Autodesk Inventor part; units mm, degrees
(part 4 of 6)
  line L2686 (41.0698, 0.537) -> (41.0192, 0.4986)
  line L2687 (41.0192, 0.4986) -> (40.9808, 0.4573)
  line L2688 (40.9808, 0.4573) -> (40.9546, 0.4142)
  line L2689 (40.9546, 0.4142) -> (40.9408, 0.3701)
  line L2690 (40.9408, 0.3701) -> (40.9386, 0.337)
  line L2691 (40.9386, 0.337) -> (40.9471, 0.1693)
  line L2692 (40.9471, 0.1693) -> (40.95, 0)
  line L2693 (40.95, 0) -> (40.9471, -0.1693)
  line L2694 (40.9471, -0.1693) -> (40.9386, -0.337)
  line L2695 (40.9386, -0.337) -> (40.9408, -0.3701)
  line L2696 (40.9408, -0.3701) -> (40.9546, -0.4142)
  line L2697 (40.9546, -0.4142) -> (40.9808, -0.4573)
  line L2698 (40.9808, -0.4573) -> (41.0192, -0.4986)
  line L2699 (41.0192, -0.4986) -> (41.0698, -0.537)
  line L2700 (41.0698, -0.537) -> (41.1323, -0.5716)
  line L2701 (41.1323, -0.5716) -> (41.2066, -0.6014)
  line L2702 (41.2066, -0.6014) -> (41.2923, -0.6256)
  line L2703 (41.2923, -0.6256) -> (41.389, -0.6433)
  line L2704 (41.389, -0.6433) -> (41.4963, -0.6535)
  line L2705 (41.4963, -0.6535) -> (41.6138, -0.6555)
  line L2706 (41.6138, -0.6555) -> (41.6635, -0.6665)
  line L2707 (41.6635, -0.6665) -> (41.7507, -0.6947)
  line L2708 (41.7507, -0.6947) -> (41.8718, -0.7452)
  line L2709 (41.8718, -0.7452) -> (41.9437, -0.7805)
  line L2710 (41.9437, -0.7805) -> (42.0233, -0.8239)
  line L2711 (42.0233, -0.8239) -> (42.1084, -0.875)
  line L2712 (42.1084, -0.875) -> (42.2012, -0.9361)
  line L2713 (42.2012, -0.9361) -> (42.2978, -1.0056)
  line L2714 (42.2978, -1.0056) -> (42.4003, -1.0861)
  line L2715 (42.4003, -1.0861) -> (42.5064, -1.177)
  line L2716 (42.5064, -1.177) -> (42.6163, -1.2793)
  line L2717 (42.6163, -1.2793) -> (42.7287, -1.3932)
  line L2718 (42.7287, -1.3932) -> (42.8351, -1.5103)
  arc A83 (42.6745, -2.1096) -> (42.8351, -1.5103) centre (36, 0) ccw
  line L2719 (42.6745, -2.1096) -> (42.5238, -2.1578)
  line L2720 (42.5238, -2.1578) -> (42.3695, -2.2002)
  line L2721 (42.3695, -2.2002) -> (42.2232, -2.2339)
  line L2722 (42.2232, -2.2339) -> (42.0859, -2.2595)
  line L2723 (42.0859, -2.2595) -> (41.9569, -2.278)
  line L2724 (41.9569, -2.278) -> (41.8384, -2.2899)
  line L2725 (41.8384, -2.2899) -> (41.7275, -2.2965)
  line L2726 (41.7275, -2.2965) -> (41.6283, -2.2981)
  line L2727 (41.6283, -2.2981) -> (41.5376, -2.2959)
  line L2728 (41.5376, -2.2959) -> (41.4578, -2.2905)
  line L2729 (41.4578, -2.2905) -> (41.3276, -2.2738)
  line L2730 (41.3276, -2.2738) -> (41.238, -2.2546)
  line L2731 (41.238, -2.2546) -> (41.1894, -2.2393)
  line L2732 (41.1894, -2.2393) -> (41.0867, -2.1822)
  line L2733 (41.0867, -2.1822) -> (40.9886, -2.1374)
  line L2734 (40.9886, -2.1374) -> (40.896, -2.1043)
  line L2735 (40.896, -2.1043) -> (40.8097, -2.0825)
  line L2736 (40.8097, -2.0825) -> (40.7305, -2.0712)
  line L2737 (40.7305, -2.0712) -> (40.659, -2.0699)
  line L2738 (40.659, -2.0699) -> (40.596, -2.0778)
  line L2739 (40.596, -2.0778) -> (40.5421, -2.0943)
  line L2740 (40.5421, -2.0943) -> (40.4979, -2.1186)
  line L2741 (40.4979, -2.1186) -> (40.4639, -2.1499)
  line L2742 (40.4639, -2.1499) -> (40.4454, -2.1774)
  line L2743 (40.4454, -2.1774) -> (40.369, -2.327)
  line L2744 (40.369, -2.327) -> (40.2868, -2.475)
  line L2745 (40.2868, -2.475) -> (40.1997, -2.6202)
  line L2746 (40.1997, -2.6202) -> (40.1084, -2.7611)
  line L2747 (40.1084, -2.7611) -> (40.0938, -2.7909)
  line L2748 (40.0938, -2.7909) -> (40.0837, -2.836)
  line L2749 (40.0837, -2.836) -> (40.0848, -2.8864)
  line L2750 (40.0848, -2.8864) -> (40.0975, -2.9414)
  line L2751 (40.0975, -2.9414) -> (40.1221, -2.9999)
  line L2752 (40.1221, -2.9999) -> (40.159, -3.0611)
  line L2753 (40.159, -3.0611) -> (40.2083, -3.1241)
  line L2754 (40.2083, -3.1241) -> (40.2704, -3.1879)
  line L2755 (40.2704, -3.1879) -> (40.3453, -3.2516)
  line L2756 (40.3453, -3.2516) -> (40.4332, -3.3141)
  line L2757 (40.4332, -3.3141) -> (40.534, -3.3746)
  line L2758 (40.534, -3.3746) -> (40.5715, -3.4089)
  line L2759 (40.5715, -3.4089) -> (40.6329, -3.477)
  line L2760 (40.6329, -3.477) -> (40.7125, -3.5813)
  line L2761 (40.7125, -3.5813) -> (40.7571, -3.6478)
  line L2762 (40.7571, -3.6478) -> (40.8044, -3.7252)
  line L2763 (40.8044, -3.7252) -> (40.8525, -3.8119)
  line L2764 (40.8525, -3.8119) -> (40.9023, -3.9112)
  line L2765 (40.9023, -3.9112) -> (40.9512, -4.0198)
  line L2766 (40.9512, -4.0198) -> (40.9997, -4.1408)
  line L2767 (40.9997, -4.1408) -> (41.0462, -4.2725)
  line L2768 (41.0462, -4.2725) -> (41.0902, -4.4161)
  line L2769 (41.0902, -4.4161) -> (41.1306, -4.5708)
  line L2770 (41.1306, -4.5708) -> (41.1642, -4.7255)
  arc A84 (40.7255, -5.1642) -> (41.1642, -4.7255) centre (36, 0) ccw
  line L2771 (40.7255, -5.1642) -> (40.5708, -5.1306)
  line L2772 (40.5708, -5.1306) -> (40.4161, -5.0902)
  line L2773 (40.4161, -5.0902) -> (40.2725, -5.0462)
  line L2774 (40.2725, -5.0462) -> (40.1408, -4.9997)
  line L2775 (40.1408, -4.9997) -> (40.0198, -4.9512)
  line L2776 (40.0198, -4.9512) -> (39.9112, -4.9023)
  line L2777 (39.9112, -4.9023) -> (39.8119, -4.8525)
  line L2778 (39.8119, -4.8525) -> (39.7252, -4.8044)
  line L2779 (39.7252, -4.8044) -> (39.6478, -4.7571)
  line L2780 (39.6478, -4.7571) -> (39.5813, -4.7125)
  line L2781 (39.5813, -4.7125) -> (39.477, -4.6329)
  line L2782 (39.477, -4.6329) -> (39.4089, -4.5715)
  line L2783 (39.4089, -4.5715) -> (39.3746, -4.534)
  line L2784 (39.3746, -4.534) -> (39.3141, -4.4332)
  line L2785 (39.3141, -4.4332) -> (39.2516, -4.3453)
  line L2786 (39.2516, -4.3453) -> (39.1879, -4.2704)
  line L2787 (39.1879, -4.2704) -> (39.1241, -4.2083)
  line L2788 (39.1241, -4.2083) -> (39.0611, -4.159)
  line L2789 (39.0611, -4.159) -> (38.9999, -4.1221)
  line L2790 (38.9999, -4.1221) -> (38.9414, -4.0975)
  line L2791 (38.9414, -4.0975) -> (38.8864, -4.0848)
  line L2792 (38.8864, -4.0848) -> (38.836, -4.0837)
  line L2793 (38.836, -4.0837) -> (38.7909, -4.0938)
  line L2794 (38.7909, -4.0938) -> (38.7611, -4.1084)
  line L2795 (38.7611, -4.1084) -> (38.6202, -4.1997)
  line L2796 (38.6202, -4.1997) -> (38.475, -4.2868)
  line L2797 (38.475, -4.2868) -> (38.327, -4.369)
  line L2798 (38.327, -4.369) -> (38.1774, -4.4454)
  line L2799 (38.1774, -4.4454) -> (38.1499, -4.4639)
  line L2800 (38.1499, -4.4639) -> (38.1186, -4.4979)
  line L2801 (38.1186, -4.4979) -> (38.0943, -4.5421)
  line L2802 (38.0943, -4.5421) -> (38.0778, -4.596)
  line L2803 (38.0778, -4.596) -> (38.0699, -4.659)
  line L2804 (38.0699, -4.659) -> (38.0712, -4.7305)
  line L2805 (38.0712, -4.7305) -> (38.0825, -4.8097)
  line L2806 (38.0825, -4.8097) -> (38.1043, -4.896)
  line L2807 (38.1043, -4.896) -> (38.1374, -4.9886)
  line L2808 (38.1374, -4.9886) -> (38.1822, -5.0867)
  line L2809 (38.1822, -5.0867) -> (38.2393, -5.1894)
  line L2810 (38.2393, -5.1894) -> (38.2546, -5.238)
  line L2811 (38.2546, -5.238) -> (38.2738, -5.3276)
  line L2812 (38.2738, -5.3276) -> (38.2905, -5.4578)
  line L2813 (38.2905, -5.4578) -> (38.2959, -5.5376)
  line L2814 (38.2959, -5.5376) -> (38.2981, -5.6283)
  line L2815 (38.2981, -5.6283) -> (38.2965, -5.7275)
  line L2816 (38.2965, -5.7275) -> (38.2899, -5.8384)
  line L2817 (38.2899, -5.8384) -> (38.278, -5.9569)
  line L2818 (38.278, -5.9569) -> (38.2595, -6.0859)
  line L2819 (38.2595, -6.0859) -> (38.2339, -6.2232)
  line L2820 (38.2339, -6.2232) -> (38.2002, -6.3695)
  line L2821 (38.2002, -6.3695) -> (38.1578, -6.5238)
  line L2822 (38.1578, -6.5238) -> (38.1096, -6.6745)
  arc A85 (37.5103, -6.8351) -> (38.1096, -6.6745) centre (36, 0) ccw
  line L2823 (37.5103, -6.8351) -> (37.3931, -6.7287)
  line L2824 (37.3931, -6.7287) -> (37.2793, -6.6163)
  line L2825 (37.2793, -6.6163) -> (37.177, -6.5064)
  line L2826 (37.177, -6.5064) -> (37.0862, -6.4003)
  line L2827 (37.0862, -6.4003) -> (37.0056, -6.2978)
  line L2828 (37.0056, -6.2978) -> (36.9361, -6.2012)
  line L2829 (36.9361, -6.2012) -> (36.875, -6.1084)
  line L2830 (36.875, -6.1084) -> (36.8239, -6.0233)
  line L2831 (36.8239, -6.0233) -> (36.7805, -5.9436)
  line L2832 (36.7805, -5.9436) -> (36.7452, -5.8718)
  line L2833 (36.7452, -5.8718) -> (36.6947, -5.7507)
  line L2834 (36.6947, -5.7507) -> (36.6665, -5.6635)
  line L2835 (36.6665, -5.6635) -> (36.6555, -5.6138)
  line L2836 (36.6555, -5.6138) -> (36.6535, -5.4963)
  line L2837 (36.6535, -5.4963) -> (36.6433, -5.389)
  line L2838 (36.6433, -5.389) -> (36.6256, -5.2923)
  line L2839 (36.6256, -5.2923) -> (36.6014, -5.2066)
  line L2840 (36.6014, -5.2066) -> (36.5716, -5.1323)
  line L2841 (36.5716, -5.1323) -> (36.537, -5.0698)
  line L2842 (36.537, -5.0698) -> (36.4986, -5.0192)
  line L2843 (36.4986, -5.0192) -> (36.4573, -4.9808)
  line L2844 (36.4573, -4.9808) -> (36.4142, -4.9546)
  line L2845 (36.4142, -4.9546) -> (36.3701, -4.9408)
  line L2846 (36.3701, -4.9408) -> (36.337, -4.9386)
  line L2847 (36.337, -4.9386) -> (36.1693, -4.9471)
  line L2848 (36.1693, -4.9471) -> (36, -4.95)
  line L2849 (36, -4.95) -> (35.8307, -4.9471)
  line L2850 (35.8307, -4.9471) -> (35.663, -4.9386)
  line L2851 (35.663, -4.9386) -> (35.6299, -4.9408)
  line L2852 (35.6299, -4.9408) -> (35.5858, -4.9546)
  line L2853 (35.5858, -4.9546) -> (35.5427, -4.9808)
  line L2854 (35.5427, -4.9808) -> (35.5014, -5.0192)
  line L2855 (35.5014, -5.0192) -> (35.463, -5.0698)
  line L2856 (35.463, -5.0698) -> (35.4284, -5.1323)
  line L2857 (35.4284, -5.1323) -> (35.3986, -5.2066)
  line L2858 (35.3986, -5.2066) -> (35.3744, -5.2923)
  line L2859 (35.3744, -5.2923) -> (35.3567, -5.389)
  line L2860 (35.3567, -5.389) -> (35.3465, -5.4963)
  line L2861 (35.3465, -5.4963) -> (35.3445, -5.6138)
  line L2862 (35.3445, -5.6138) -> (35.3335, -5.6635)
  line L2863 (35.3335, -5.6635) -> (35.3053, -5.7507)
  line L2864 (35.3053, -5.7507) -> (35.2548, -5.8718)
  line L2865 (35.2548, -5.8718) -> (35.2195, -5.9436)
  line L2866 (35.2195, -5.9436) -> (35.1761, -6.0233)
  line L2867 (35.1761, -6.0233) -> (35.125, -6.1084)
  line L2868 (35.125, -6.1084) -> (35.0639, -6.2012)
  line L2869 (35.0639, -6.2012) -> (34.9944, -6.2978)
  line L2870 (34.9944, -6.2978) -> (34.9138, -6.4003)
  line L2871 (34.9138, -6.4003) -> (34.823, -6.5064)
  line L2872 (34.823, -6.5064) -> (34.7207, -6.6163)
  line L2873 (34.7207, -6.6163) -> (34.6069, -6.7287)
  line L2874 (34.6069, -6.7287) -> (34.4897, -6.8351)
  arc A86 (33.8904, -6.6745) -> (34.4897, -6.8351) centre (36, 0) ccw
  line L2875 (33.8904, -6.6745) -> (33.8422, -6.5238)
  line L2876 (33.8422, -6.5238) -> (33.7998, -6.3695)
  line L2877 (33.7998, -6.3695) -> (33.7661, -6.2232)
  line L2878 (33.7661, -6.2232) -> (33.7405, -6.0859)
  line L2879 (33.7405, -6.0859) -> (33.722, -5.9569)
  line L2880 (33.722, -5.9569) -> (33.7101, -5.8384)
  line L2881 (33.7101, -5.8384) -> (33.7035, -5.7275)
  line L2882 (33.7035, -5.7275) -> (33.7019, -5.6283)
  line L2883 (33.7019, -5.6283) -> (33.7041, -5.5376)
  line L2884 (33.7041, -5.5376) -> (33.7095, -5.4578)
  line L2885 (33.7095, -5.4578) -> (33.7262, -5.3276)
  line L2886 (33.7262, -5.3276) -> (33.7454, -5.238)
  line L2887 (33.7454, -5.238) -> (33.7607, -5.1894)
  line L2888 (33.7607, -5.1894) -> (33.8178, -5.0867)
  line L2889 (33.8178, -5.0867) -> (33.8626, -4.9886)
  line L2890 (33.8626, -4.9886) -> (33.8957, -4.896)
  line L2891 (33.8957, -4.896) -> (33.9175, -4.8097)
  line L2892 (33.9175, -4.8097) -> (33.9288, -4.7305)
  line L2893 (33.9288, -4.7305) -> (33.9301, -4.659)
  line L2894 (33.9301, -4.659) -> (33.9222, -4.596)
  line L2895 (33.9222, -4.596) -> (33.9057, -4.5421)
  line L2896 (33.9057, -4.5421) -> (33.8814, -4.4979)
  line L2897 (33.8814, -4.4979) -> (33.8501, -4.4639)
  line L2898 (33.8501, -4.4639) -> (33.8226, -4.4454)
  line L2899 (33.8226, -4.4454) -> (33.673, -4.369)
  line L2900 (33.673, -4.369) -> (33.525, -4.2868)
  line L2901 (33.525, -4.2868) -> (33.3798, -4.1997)
  line L2902 (33.3798, -4.1997) -> (33.2389, -4.1084)
  line L2903 (33.2389, -4.1084) -> (33.2091, -4.0938)
  line L2904 (33.2091, -4.0938) -> (33.164, -4.0837)
  line L2905 (33.164, -4.0837) -> (33.1136, -4.0848)
  line L2906 (33.1136, -4.0848) -> (33.0586, -4.0975)
  line L2907 (33.0586, -4.0975) -> (33.0001, -4.1221)
  line L2908 (33.0001, -4.1221) -> (32.9389, -4.159)
  line L2909 (32.9389, -4.159) -> (32.8759, -4.2083)
  line L2910 (32.8759, -4.2083) -> (32.8121, -4.2704)
  line L2911 (32.8121, -4.2704) -> (32.7484, -4.3453)
  line L2912 (32.7484, -4.3453) -> (32.6859, -4.4332)
  line L2913 (32.6859, -4.4332) -> (32.6254, -4.534)
  line L2914 (32.6254, -4.534) -> (32.5911, -4.5715)
  line L2915 (32.5911, -4.5715) -> (32.523, -4.6329)
  line L2916 (32.523, -4.6329) -> (32.4187, -4.7125)
  line L2917 (32.4187, -4.7125) -> (32.3522, -4.7571)
  line L2918 (32.3522, -4.7571) -> (32.2748, -4.8044)
  line L2919 (32.2748, -4.8044) -> (32.1881, -4.8525)
  line L2920 (32.1881, -4.8525) -> (32.0888, -4.9023)
  line L2921 (32.0888, -4.9023) -> (31.9802, -4.9512)
  line L2922 (31.9802, -4.9512) -> (31.8592, -4.9997)
  line L2923 (31.8592, -4.9997) -> (31.7275, -5.0462)
  line L2924 (31.7275, -5.0462) -> (31.5839, -5.0902)
  line L2925 (31.5839, -5.0902) -> (31.4292, -5.1306)
  line L2926 (31.4292, -5.1306) -> (31.2745, -5.1642)
  arc A87 (30.8358, -4.7255) -> (31.2745, -5.1642) centre (36, 0) ccw
  line L2927 (30.8358, -4.7255) -> (30.8694, -4.5708)
  line L2928 (30.676, 2.741) -> (30.453, 2.6211)
  line L2929 (30.453, 2.6211) -> (30.2376, 2.5111)
  line L2930 (30.2376, 2.5111) -> (30.0323, 2.4116)
  line L2931 (30.0323, 2.4116) -> (29.8355, 2.3213)
  line L2932 (29.8355, 2.3213) -> (29.6473, 2.2396)
  line L2933 (29.6473, 2.2396) -> (29.4705, 2.1673)
  line L2934 (29.4705, 2.1673) -> (29.3033, 2.1029)
  line L2935 (29.3033, 2.1029) -> (28.9724, 1.9849)
  line L2936 (28.9724, 1.9849) -> (28.931, 1.9629)
  line L2937 (28.931, 1.9629) -> (28.9033, 1.9404)
  line L2938 (28.9033, 1.9404) -> (28.8892, 1.9178)
  line L2939 (28.8892, 1.9178) -> (28.8876, 1.9012)
  line L2940 (28.8876, 1.9012) -> (28.9103, 1.5151)
  line L2941 (28.9103, 1.5151) -> (28.9281, 1.1288)
  line L2942 (28.9281, 1.1288) -> (28.9314, 1.1124)
  line L2943 (28.9314, 1.1124) -> (28.9478, 1.0915)
  line L2944 (28.9478, 1.0915) -> (28.9777, 1.0719)
  line L2945 (28.9777, 1.0719) -> (29.0211, 1.0544)
  line L2946 (29.0211, 1.0544) -> (29.3626, 0.9717)
  line L2947 (29.3626, 0.9717) -> (29.5356, 0.9251)
  line L2948 (29.5356, 0.9251) -> (29.719, 0.8717)
  line L2949 (29.719, 0.8717) -> (29.9147, 0.8101)
  line L2950 (29.9147, 0.8101) -> (30.1199, 0.7408)
  line L2951 (30.1199, 0.7408) -> (30.3344, 0.6634)
  line L2952 (30.3344, 0.6634) -> (30.5601, 0.5765)
  line L2953 (30.5601, 0.5765) -> (30.7945, 0.4805)
  line L2954 (30.7945, 0.4805) -> (30.9975, 0.3928)
  arc A88 (30.9975, -0.3928) -> (30.9975, 0.3928) centre (0, 0) ccw
  line L2955 (30.9975, -0.3928) -> (30.7945, -0.4805)
  line L2956 (30.7945, -0.4805) -> (30.5601, -0.5765)
  line L2957 (30.5601, -0.5765) -> (30.3344, -0.6634)
  line L2958 (30.3344, -0.6634) -> (30.1199, -0.7408)
  line L2959 (30.1199, -0.7408) -> (29.9147, -0.8101)
  line L2960 (29.9147, -0.8101) -> (29.719, -0.8717)
  line L2961 (29.719, -0.8717) -> (29.5356, -0.9251)
  line L2962 (29.5356, -0.9251) -> (29.3626, -0.9717)
  line L2963 (29.3626, -0.9717) -> (29.0211, -1.0544)
  line L2964 (29.0211, -1.0544) -> (28.9777, -1.0719)
  line L2965 (28.9777, -1.0719) -> (28.9478, -1.0915)
  line L2966 (28.9478, -1.0915) -> (28.9314, -1.1124)
  line L2967 (28.9314, -1.1124) -> (28.9281, -1.1288)
  line L2968 (28.9281, -1.1288) -> (28.9103, -1.5151)
  line L2969 (28.9103, -1.5151) -> (28.8876, -1.9012)
  line L2970 (28.8876, -1.9012) -> (28.8892, -1.9178)
  line L2971 (28.8892, -1.9178) -> (28.9033, -1.9404)
  line L2972 (28.9033, -1.9404) -> (28.931, -1.9629)
  line L2973 (28.931, -1.9629) -> (28.9724, -1.9849)
  line L2974 (28.9724, -1.9849) -> (29.3033, -2.1029)
  line L2975 (29.3033, -2.1029) -> (29.4705, -2.1673)
  line L2976 (29.4705, -2.1673) -> (29.6473, -2.2396)
  line L2977 (29.6473, -2.2396) -> (29.8355, -2.3213)
  line L2978 (29.8355, -2.3213) -> (30.0323, -2.4116)
  line L2979 (30.0323, -2.4116) -> (30.2376, -2.5111)
  line L2980 (30.2376, -2.5111) -> (30.453, -2.6211)
  line L2981 (30.453, -2.6211) -> (30.676, -2.741)
  line L2982 (30.676, -2.741) -> (30.8688, -2.8495)
  arc A89 (30.7866, -3.6308) -> (30.8688, -2.8495) centre (0, 0) ccw
  line L2983 (30.7866, -3.6308) -> (30.5755, -3.6968)
  line L2984 (30.5755, -3.6968) -> (30.3325, -3.7677)
  line L2985 (30.3325, -3.7677) -> (30.0989, -3.8305)
  line L2986 (30.0989, -3.8305) -> (29.8774, -3.8852)
  line L2987 (29.8774, -3.8852) -> (29.6661, -3.9326)
  line L2988 (29.6661, -3.9326) -> (29.465, -3.9734)
  line L2989 (29.465, -3.9734) -> (29.2771, -4.0074)
  line L2990 (29.2771, -4.0074) -> (29.1001, -4.0356)
  line L2991 (29.1001, -4.0356) -> (28.7519, -4.0822)
  line L2992 (28.7519, -4.0822) -> (28.7069, -4.0951)
  line L2993 (28.7069, -4.0951) -> (28.6751, -4.1114)
  line L2994 (28.6751, -4.1114) -> (28.6567, -4.1305)
  line L2995 (28.6567, -4.1305) -> (28.6516, -4.1464)
  line L2996 (28.6516, -4.1464) -> (28.5936, -4.5288)
  line L2997 (28.5936, -4.5288) -> (28.5306, -4.9104)
  line L2998 (28.5306, -4.9104) -> (28.5305, -4.927)
  line L2999 (28.5305, -4.927) -> (28.5421, -4.951)
  line L3000 (28.5421, -4.951) -> (28.5674, -4.9763)
  line L3001 (28.5674, -4.9763) -> (28.6062, -5.0025)
  line L3002 (28.6062, -5.0025) -> (28.9229, -5.1544)
  line L3003 (28.9229, -5.1544) -> (29.0826, -5.2359)
  line L3004 (29.0826, -5.2359) -> (29.2508, -5.3263)
  line L3005 (29.2508, -5.3263) -> (29.4294, -5.4272)
  line L3006 (29.4294, -5.4272) -> (29.6157, -5.5376)
  line L3007 (29.6157, -5.5376) -> (29.8094, -5.658)
  line L3008 (29.8094, -5.658) -> (30.0122, -5.79)
  line L3009 (30.0122, -5.79) -> (30.2214, -5.9325)
  line L3010 (30.2214, -5.9325) -> (30.4018, -6.0605)
  arc A90 (30.2385, -6.829) -> (30.4018, -6.0605) centre (0, 0) ccw
  line L3011 (30.2385, -6.829) -> (30.0216, -6.8726)
  line L3012 (30.0216, -6.8726) -> (29.7725, -6.9177)
  line L3013 (29.7725, -6.9177) -> (29.5336, -6.9557)
  line L3014 (29.5336, -6.9557) -> (29.3077, -6.9869)
  line L3015 (29.3077, -6.9869) -> (29.0926, -7.012)
  line L3016 (29.0926, -7.012) -> (28.8883, -7.0315)
  line L3017 (28.8883, -7.0315) -> (28.6979, -7.0457)
  line L3018 (28.6979, -7.0457) -> (28.5189, -7.0553)
  line L3019 (28.5189, -7.0553) -> (28.1677, -7.0652)
  line L3020 (28.1677, -7.0652) -> (28.1216, -7.0733)
  line L3021 (28.1216, -7.0733) -> (28.0883, -7.0862)
  line L3022 (28.0883, -7.0862) -> (28.0679, -7.1033)
  line L3023 (28.0679, -7.1033) -> (28.0612, -7.1186)
  line L3024 (28.0612, -7.1186) -> (27.9636, -7.4928)
  line L3025 (27.9636, -7.4928) -> (27.861, -7.8657)
  line L3026 (27.861, -7.8657) -> (27.8592, -7.8823)
  line L3027 (27.8592, -7.8823) -> (27.8683, -7.9073)
  line L3028 (27.8683, -7.9073) -> (27.8907, -7.9351)
  line L3029 (27.8907, -7.9351) -> (27.9266, -7.9652)
  line L3030 (27.9266, -7.9652) -> (28.2257, -8.1494)
  line L3031 (28.2257, -8.1494) -> (28.3759, -8.2472)
  line L3032 (28.3759, -8.2472) -> (28.5338, -8.3547)
  line L3033 (28.5338, -8.3547) -> (28.7009, -8.4737)
  line L3034 (28.7009, -8.4737) -> (28.8746, -8.603)
  line L3035 (28.8746, -8.603) -> (29.0547, -8.7429)
  line L3036 (29.0547, -8.7429) -> (29.2425, -8.8954)
  line L3037 (29.2425, -8.8954) -> (29.4358, -9.059)
  line L3038 (29.4358, -9.059) -> (29.6018, -9.2052)
  arc A91 (29.359, -9.9523) -> (29.6018, -9.2052) centre (0, 0) ccw
  line L3039 (29.359, -9.9523) -> (29.1388, -9.973)
  line L3040 (29.1388, -9.973) -> (28.8863, -9.9918)
  line L3041 (28.8863, -9.9918) -> (28.6447, -10.0047)
  line L3042 (28.6447, -10.0047) -> (28.4168, -10.0121)
  line L3043 (28.4168, -10.0121) -> (28.2002, -10.0146)
  line L3044 (28.2002, -10.0146) -> (27.995, -10.0127)
  line L3045 (27.995, -10.0127) -> (27.8042, -10.0069)
  line L3046 (27.8042, -10.0069) -> (27.6252, -9.9977)
  line L3047 (27.6252, -9.9977) -> (27.2749, -9.9708)
  line L3048 (27.2749, -9.9708) -> (27.2282, -9.9741)
  line L3049 (27.2282, -9.9741) -> (27.1937, -9.9834)
  line L3050 (27.1937, -9.9834) -> (27.1717, -9.9983)
  line L3051 (27.1717, -9.9983) -> (27.1634, -10.0128)
  line L3052 (27.1634, -10.0128) -> (27.0272, -10.3748)
  line L3053 (27.0272, -10.3748) -> (26.8862, -10.7349)
  line L3054 (26.8862, -10.7349) -> (26.8826, -10.7512)
  line L3055 (26.8826, -10.7512) -> (26.8891, -10.777)
  line L3056 (26.8891, -10.777) -> (26.9085, -10.807)
  line L3057 (26.9085, -10.807) -> (26.941, -10.8407)
  line L3058 (26.941, -10.8407) -> (27.2193, -11.0551)
  line L3059 (27.2193, -11.0551) -> (27.3584, -11.1681)
  line L3060 (27.3584, -11.1681) -> (27.5042, -11.2915)
  line L3061 (27.5042, -11.2915) -> (27.6579, -11.4273)
  line L3062 (27.6579, -11.4273) -> (27.8172, -11.5741)
  line L3063 (27.8172, -11.5741) -> (27.9817, -11.7321)
  line L3064 (27.9817, -11.7321) -> (28.1525, -11.9033)
  line L3065 (28.1525, -11.9033) -> (28.3276, -12.0862)
  line L3066 (28.3276, -12.0862) -> (28.4774, -12.249)
  arc A92 (28.1579, -12.9667) -> (28.4774, -12.249) centre (0, 0) ccw
  line L3067 (28.1579, -12.9667) -> (27.9367, -12.9642)
  line L3068 (27.9367, -12.9642) -> (27.6836, -12.9565)
  line L3069 (27.6836, -12.9565) -> (27.442, -12.9441)
  line L3070 (27.442, -12.9441) -> (27.2145, -12.9276)
  line L3071 (27.2145, -12.9276) -> (26.9989, -12.9075)
  line L3072 (26.9989, -12.9075) -> (26.7951, -12.8841)
  line L3073 (26.7951, -12.8841) -> (26.6059, -12.8584)
  line L3074 (26.6059, -12.8584) -> (26.4288, -12.8305)
  line L3075 (26.4288, -12.8305) -> (26.0833, -12.7672)
  line L3076 (26.0833, -12.7672) -> (26.0365, -12.7656)
  line L3077 (26.0365, -12.7656) -> (26.0012, -12.7712)
  line L3078 (26.0012, -12.7712) -> (25.9777, -12.7837)
  line L3079 (25.9777, -12.7837) -> (25.968, -12.7973)
  line L3080 (25.968, -12.7973) -> (25.7946, -13.143)
  line L3081 (25.7946, -13.143) -> (25.6168, -13.4865)
  line L3082 (25.6168, -13.4865) -> (25.6116, -13.5023)
  line L3083 (25.6116, -13.5023) -> (25.6153, -13.5287)
  line L3084 (25.6153, -13.5287) -> (25.6314, -13.5605)
  line L3085 (25.6314, -13.5605) -> (25.6603, -13.5974)
  line L3086 (25.6603, -13.5974) -> (25.9146, -13.8398)
  line L3087 (25.9146, -13.8398) -> (26.0412, -13.9666)
  line L3088 (26.0412, -13.9666) -> (26.1732, -14.1046)
  line L3089 (26.1732, -14.1046) -> (26.312, -14.2558)
  line L3090 (26.312, -14.2558) -> (26.455, -14.4184)
  line L3091 (26.455, -14.4184) -> (26.602, -14.5927)
  line L3092 (26.602, -14.5927) -> (26.7541, -14.7808)
  line L3093 (26.7541, -14.7808) -> (26.9091, -14.9811)
  line L3094 (26.9091, -14.9811) -> (27.041, -15.1586)
  arc A93 (26.6482, -15.8389) -> (27.041, -15.1586) centre (0, 0) ccw
  line L3095 (26.6482, -15.8389) -> (26.4285, -15.8134)
  line L3096 (26.4285, -15.8134) -> (26.1776, -15.7793)
  line L3097 (26.1776, -15.7793) -> (25.9387, -15.7417)
  line L3098 (25.9387, -15.7417) -> (25.7142, -15.7015)
  line L3099 (25.7142, -15.7015) -> (25.5018, -15.6589)
  line L3100 (25.5018, -15.6589) -> (25.3015, -15.6144)
  line L3101 (25.3015, -15.6144) -> (25.1161, -15.569)
  line L3102 (25.1161, -15.569) -> (24.9429, -15.5228)
  line L3103 (24.9429, -15.5228) -> (24.6058, -15.4237)
  line L3104 (24.6058, -15.4237) -> (24.5595, -15.4172)
  line L3105 (24.5595, -15.4172) -> (24.5238, -15.4191)
  line L3106 (24.5238, -15.4191) -> (24.4991, -15.4291)
  line L3107 (24.4991, -15.4291) -> (24.488, -15.4416)
  line L3108 (24.488, -15.4416) -> (24.2795, -15.7673)
  line L3109 (24.2795, -15.7673) -> (24.0668, -16.0903)
  line L3110 (24.0668, -16.0903) -> (24.0599, -16.1055)
  line L3111 (24.0599, -16.1055) -> (24.0608, -16.1321)
  line L3112 (24.0608, -16.1321) -> (24.0735, -16.1655)
  line L3113 (24.0735, -16.1655) -> (24.0984, -16.2052)
  line L3114 (24.0984, -16.2052) -> (24.326, -16.4728)
  line L3115 (24.326, -16.4728) -> (24.4386, -16.6122)
  line L3116 (24.4386, -16.6122) -> (24.5555, -16.7632)
  line L3117 (24.5555, -16.7632) -> (24.6777, -16.928)
  line L3118 (24.6777, -16.928) -> (24.8029, -17.1047)
  line L3119 (24.8029, -17.1047) -> (24.931, -17.2934)
  line L3120 (24.931, -17.2934) -> (25.0625, -17.4964)
  line L3121 (25.0625, -17.4964) -> (25.1957, -17.7118)
  line L3122 (25.1957, -17.7118) -> (25.3084, -17.9021)
  arc A94 (24.8466, -18.5377) -> (25.3084, -17.9021) centre (0, 0) ccw
  line L3123 (24.8466, -18.5377) -> (24.6308, -18.4893)
  line L3124 (24.6308, -18.4893) -> (24.3848, -18.4292)
  line L3125 (24.3848, -18.4292) -> (24.1511, -18.3668)
  line L3126 (24.1511, -18.3668) -> (23.932, -18.3034)
  line L3127 (23.932, -18.3034) -> (23.7253, -18.2388)
  line L3128 (23.7253, -18.2388) -> (23.5308, -18.1736)
  line L3129 (23.5308, -18.1736) -> (23.3511, -18.1091)
  line L3130 (23.3511, -18.1091) -> (23.1837, -18.045)
  line L3131 (23.1837, -18.045) -> (22.8588, -17.9112)
  line L3132 (22.8588, -17.9112) -> (22.8134, -17.8999)
  line L3133 (22.8134, -17.8999) -> (22.7777, -17.8981)
  line L3134 (22.7777, -17.8981) -> (22.7521, -17.9055)
  line L3135 (22.7521, -17.9055) -> (22.7398, -17.9167)
  line L3136 (22.7398, -17.9167) -> (22.4984, -18.2188)
  line L3137 (22.4984, -18.2188) -> (22.2531, -18.5178)
  line L3138 (22.2531, -18.5178) -> (22.2446, -18.5322)
  line L3139 (22.2446, -18.5322) -> (22.2427, -18.5587)
  line L3140 (22.2427, -18.5587) -> (22.2519, -18.5933)
  line L3141 (22.2519, -18.5933) -> (22.2724, -18.6353)
  line L3142 (22.2724, -18.6353) -> (22.4708, -18.9253)
  line L3143 (22.4708, -18.9253) -> (22.5683, -19.0757)
  line L3144 (22.5683, -19.0757) -> (22.6688, -19.2381)
  line L3145 (22.6688, -19.2381) -> (22.773, -19.4148)
  line L3146 (22.773, -19.4148) -> (22.8791, -19.6036)
  line L3147 (22.8791, -19.6036) -> (22.9867, -19.8047)
  line L3148 (22.9867, -19.8047) -> (23.0963, -20.0203)
  line L3149 (23.0963, -20.0203) -> (23.2063, -20.2484)
  line L3150 (23.2063, -20.2484) -> (23.2985, -20.4495)
  arc A95 (22.7728, -21.0333) -> (23.2985, -20.4495) centre (0, 0) ccw
  line L3151 (22.7728, -21.0333) -> (22.5632, -20.9626)
  line L3152 (22.5632, -20.9626) -> (22.3249, -20.8771)
  line L3153 (22.3249, -20.8771) -> (22.099, -20.7906)
  line L3154 (22.099, -20.7906) -> (21.8877, -20.7047)
  line L3155 (21.8877, -20.7047) -> (21.6889, -20.6189)
  line L3156 (21.6889, -20.6189) -> (21.5022, -20.5336)
  line L3157 (21.5022, -20.5336) -> (21.3302, -20.4507)
  line L3158 (21.3302, -20.4507) -> (21.1705, -20.3695)
  line L3159 (21.1705, -20.3695) -> (20.8614, -20.2025)
  line L3160 (20.8614, -20.2025) -> (20.8174, -20.1865)
  line L3161 (20.8174, -20.1865) -> (20.7821, -20.181)
  line L3162 (20.7821, -20.181) -> (20.7559, -20.1856)
  line L3163 (20.7559, -20.1856) -> (20.7424, -20.1955)
  line L3164 (20.7424, -20.1955) -> (20.4707, -20.4707)
  line L3165 (20.4707, -20.4707) -> (20.1955, -20.7424)
  line L3166 (20.1955, -20.7424) -> (20.1856, -20.7559)
  line L3167 (20.1856, -20.7559) -> (20.181, -20.7821)
  line L3168 (20.181, -20.7821) -> (20.1865, -20.8174)
  line L3169 (20.1865, -20.8174) -> (20.2025, -20.8614)
  line L3170 (20.2025, -20.8614) -> (20.3695, -21.1705)
  line L3171 (20.3695, -21.1705) -> (20.4507, -21.3302)
  line L3172 (20.4507, -21.3302) -> (20.5336, -21.5022)
  line L3173 (20.5336, -21.5022) -> (20.6189, -21.6889)
  line L3174 (20.6189, -21.6889) -> (20.7047, -21.8877)
  line L3175 (20.7047, -21.8877) -> (20.7906, -22.099)
  line L3176 (20.7906, -22.099) -> (20.8771, -22.3249)
  line L3177 (20.8771, -22.3249) -> (20.9626, -22.5632)
  line L3178 (20.9626, -22.5632) -> (21.0333, -22.7728)
  arc A96 (20.4495, -23.2985) -> (21.0333, -22.7728) centre (0, 0) ccw
  line L3179 (20.4495, -23.2985) -> (20.2484, -23.2063)
  line L3180 (20.2484, -23.2063) -> (20.0203, -23.0963)
  line L3181 (20.0203, -23.0963) -> (19.8047, -22.9867)
  line L3182 (19.8047, -22.9867) -> (19.6036, -22.8791)
  line L3183 (19.6036, -22.8791) -> (19.4148, -22.773)
  line L3184 (19.4148, -22.773) -> (19.2381, -22.6688)
  line L3185 (19.2381, -22.6688) -> (19.0757, -22.5683)
  line L3186 (19.0757, -22.5683) -> (18.9253, -22.4708)
  line L3187 (18.9253, -22.4708) -> (18.6353, -22.2724)
  line L3188 (18.6353, -22.2724) -> (18.5933, -22.2519)
  line L3189 (18.5933, -22.2519) -> (18.5587, -22.2427)
  line L3190 (18.5587, -22.2427) -> (18.5322, -22.2446)
  line L3191 (18.5322, -22.2446) -> (18.5178, -22.2531)
  line L3192 (18.5178, -22.2531) -> (18.2188, -22.4984)
  line L3193 (18.2188, -22.4984) -> (17.9167, -22.7398)
  line L3194 (17.9167, -22.7398) -> (17.9055, -22.7521)
  line L3195 (17.9055, -22.7521) -> (17.8981, -22.7777)
  line L3196 (17.8981, -22.7777) -> (17.8999, -22.8134)
  line L3197 (17.8999, -22.8134) -> (17.9112, -22.8588)
  line L3198 (17.9112, -22.8588) -> (18.045, -23.1837)
  line L3199 (18.045, -23.1837) -> (18.1091, -23.3511)
  line L3200 (18.1091, -23.3511) -> (18.1736, -23.5308)
  line L3201 (18.1736, -23.5308) -> (18.2388, -23.7253)
  line L3202 (18.2388, -23.7253) -> (18.3034, -23.932)
  line L3203 (18.3034, -23.932) -> (18.3668, -24.1511)
  line L3204 (18.3668, -24.1511) -> (18.4292, -24.3848)
  line L3205 (18.4292, -24.3848) -> (18.4893, -24.6308)
  line L3206 (18.4893, -24.6308) -> (18.5377, -24.8466)
  arc A97 (17.9021, -25.3084) -> (18.5377, -24.8466) centre (0, 0) ccw
  line L3207 (17.9021, -25.3084) -> (17.7118, -25.1957)
  line L3208 (17.7118, -25.1957) -> (17.4964, -25.0625)
  line L3209 (17.4964, -25.0625) -> (17.2934, -24.931)
  line L3210 (17.2934, -24.931) -> (17.1047, -24.8029)
  line L3211 (17.1047, -24.8029) -> (16.928, -24.6777)
  line L3212 (16.928, -24.6777) -> (16.7632, -24.5555)
  line L3213 (16.7632, -24.5555) -> (16.6122, -24.4386)
  line L3214 (16.6122, -24.4386) -> (16.4728, -24.326)
  line L3215 (16.4728, -24.326) -> (16.2052, -24.0984)
  line L3216 (16.2052, -24.0984) -> (16.1655, -24.0735)
  line L3217 (16.1655, -24.0735) -> (16.1321, -24.0608)
  line L3218 (16.1321, -24.0608) -> (16.1055, -24.0599)
  line L3219 (16.1055, -24.0599) -> (16.0903, -24.0668)
  line L3220 (16.0903, -24.0668) -> (15.7673, -24.2795)
  line L3221 (15.7673, -24.2795) -> (15.4416, -24.488)
  line L3222 (15.4416, -24.488) -> (15.4291, -24.4991)
  line L3223 (15.4291, -24.4991) -> (15.4191, -24.5238)
  line L3224 (15.4191, -24.5238) -> (15.4172, -24.5595)
  line L3225 (15.4172, -24.5595) -> (15.4237, -24.6058)
  line L3226 (15.4237, -24.6058) -> (15.5228, -24.9429)
  line L3227 (15.5228, -24.9429) -> (15.569, -25.1161)
  line L3228 (15.569, -25.1161) -> (15.6144, -25.3015)
  line L3229 (15.6144, -25.3015) -> (15.6589, -25.5018)
  line L3230 (15.6589, -25.5018) -> (15.7015, -25.7142)
  line L3231 (15.7015, -25.7142) -> (15.7417, -25.9387)
  line L3232 (15.7417, -25.9387) -> (15.7793, -26.1776)
  line L3233 (15.7793, -26.1776) -> (15.8134, -26.4285)
  line L3234 (15.8134, -26.4285) -> (15.8389, -26.6482)
  arc A98 (15.1586, -27.041) -> (15.8389, -26.6482) centre (0, 0) ccw
  line L3235 (15.1586, -27.041) -> (14.9811, -26.9091)
  line L3236 (14.9811, -26.9091) -> (14.7808, -26.7541)
  line L3237 (14.7808, -26.7541) -> (14.5927, -26.602)
  line L3238 (14.5927, -26.602) -> (14.4184, -26.455)
  line L3239 (14.4184, -26.455) -> (14.2558, -26.312)
  line L3240 (14.2558, -26.312) -> (14.1046, -26.1732)
  line L3241 (14.1046, -26.1732) -> (13.9666, -26.0412)
  line L3242 (13.9666, -26.0412) -> (13.8398, -25.9146)
  line L3243 (13.8398, -25.9146) -> (13.5974, -25.6603)
  line L3244 (13.5974, -25.6603) -> (13.5605, -25.6314)
  line L3245 (13.5605, -25.6314) -> (13.5287, -25.6153)
  line L3246 (13.5287, -25.6153) -> (13.5023, -25.6116)
  line L3247 (13.5023, -25.6116) -> (13.4865, -25.6168)
  line L3248 (13.4865, -25.6168) -> (13.143, -25.7946)
  line L3249 (13.143, -25.7946) -> (12.7973, -25.968)
  line L3250 (12.7973, -25.968) -> (12.7837, -25.9777)
  line L3251 (12.7837, -25.9777) -> (12.7712, -26.0012)
  line L3252 (12.7712, -26.0012) -> (12.7656, -26.0365)
  line L3253 (12.7656, -26.0365) -> (12.7672, -26.0833)
  line L3254 (12.7672, -26.0833) -> (12.8305, -26.4288)
  line L3255 (12.8305, -26.4288) -> (12.8584, -26.6059)
  line L3256 (12.8584, -26.6059) -> (12.8841, -26.7951)
  line L3257 (12.8841, -26.7951) -> (12.9075, -26.9989)
  line L3258 (12.9075, -26.9989) -> (12.9276, -27.2145)
  line L3259 (12.9276, -27.2145) -> (12.9441, -27.442)
  line L3260 (12.9441, -27.442) -> (12.9565, -27.6836)
  line L3261 (12.9565, -27.6836) -> (12.9642, -27.9367)
  line L3262 (12.9642, -27.9367) -> (12.9667, -28.1579)
  arc A99 (12.249, -28.4774) -> (12.9667, -28.1579) centre (0, 0) ccw
  line L3263 (12.249, -28.4774) -> (12.0862, -28.3276)
  line L3264 (12.0862, -28.3276) -> (11.9033, -28.1525)
  line L3265 (11.9033, -28.1525) -> (11.7321, -27.9817)
  line L3266 (11.7321, -27.9817) -> (11.5741, -27.8172)
  line L3267 (11.5741, -27.8172) -> (11.4273, -27.6579)
  line L3268 (11.4273, -27.6579) -> (11.2915, -27.5042)
  line L3269 (11.2915, -27.5042) -> (11.1681, -27.3584)
  line L3270 (11.1681, -27.3584) -> (11.0551, -27.2193)
  line L3271 (11.0551, -27.2193) -> (10.8407, -26.941)
  line L3272 (10.8407, -26.941) -> (10.807, -26.9085)
  line L3273 (10.807, -26.9085) -> (10.777, -26.8891)
  line L3274 (10.777, -26.8891) -> (10.7512, -26.8826)
  line L3275 (10.7512, -26.8826) -> (10.7349, -26.8862)
  line L3276 (10.7349, -26.8862) -> (10.3748, -27.0272)
  line L3277 (10.3748, -27.0272) -> (10.0128, -27.1634)
  line L3278 (10.0128, -27.1634) -> (9.9983, -27.1717)
  line L3279 (9.9983, -27.1717) -> (9.9834, -27.1937)
  line L3280 (9.9834, -27.1937) -> (9.9741, -27.2282)
  line L3281 (9.9741, -27.2282) -> (9.9708, -27.2749)
  line L3282 (9.9708, -27.2749) -> (9.9977, -27.6252)
  line L3283 (9.9977, -27.6252) -> (10.0069, -27.8042)
  line L3284 (10.0069, -27.8042) -> (10.0127, -27.995)
  line L3285 (10.0127, -27.995) -> (10.0146, -28.2002)
  line L3286 (10.0146, -28.2002) -> (10.0121, -28.4168)
  line L3287 (10.0121, -28.4168) -> (10.0047, -28.6447)
  line L3288 (10.0047, -28.6447) -> (9.9918, -28.8863)
  line L3289 (9.9918, -28.8863) -> (9.973, -29.1388)
  line L3290 (9.973, -29.1388) -> (9.9523, -29.359)
  arc A100 (9.2052, -29.6018) -> (9.9523, -29.359) centre (0, 0) ccw
  line L3291 (9.2052, -29.6018) -> (9.059, -29.4358)
  line L3292 (9.059, -29.4358) -> (8.8954, -29.2425)
  line L3293 (8.8954, -29.2425) -> (8.7429, -29.0547)
  line L3294 (8.7429, -29.0547) -> (8.603, -28.8746)
  line L3295 (8.603, -28.8746) -> (8.4737, -28.7009)
  line L3296 (8.4737, -28.7009) -> (8.3547, -28.5338)
  line L3297 (8.3547, -28.5338) -> (8.2472, -28.3759)
  line L3298 (8.2472, -28.3759) -> (8.1494, -28.2257)
  line L3299 (8.1494, -28.2257) -> (7.9652, -27.9266)
  line L3300 (7.9652, -27.9266) -> (7.9351, -27.8907)
  line L3301 (7.9351, -27.8907) -> (7.9073, -27.8683)
  line L3302 (7.9073, -27.8683) -> (7.8823, -27.8592)
  line L3303 (7.8823, -27.8592) -> (7.8657, -27.861)
  line L3304 (7.8657, -27.861) -> (7.4928, -27.9636)
  line L3305 (7.4928, -27.9636) -> (7.1186, -28.0612)
  line L3306 (7.1186, -28.0612) -> (7.1033, -28.0679)
  line L3307 (7.1033, -28.0679) -> (7.0862, -28.0883)
  line L3308 (7.0862, -28.0883) -> (7.0733, -28.1216)
  line L3309 (7.0733, -28.1216) -> (7.0652, -28.1677)
  line L3310 (7.0652, -28.1677) -> (7.0553, -28.5189)
  line L3311 (7.0553, -28.5189) -> (7.0457, -28.6979)
  line L3312 (7.0457, -28.6979) -> (7.0315, -28.8883)
  line L3313 (7.0315, -28.8883) -> (7.012, -29.0926)
  line L3314 (7.012, -29.0926) -> (6.9869, -29.3077)
  line L3315 (6.9869, -29.3077) -> (6.9557, -29.5336)
  line L3316 (6.9557, -29.5336) -> (6.9177, -29.7725)
  line L3317 (6.9177, -29.7725) -> (6.8726, -30.0216)
  line L3318 (6.8726, -30.0216) -> (6.829, -30.2385)
  arc A101 (6.0605, -30.4018) -> (6.829, -30.2385) centre (0, 0) ccw
  line L3319 (6.0605, -30.4018) -> (5.9325, -30.2214)
  line L3320 (5.9325, -30.2214) -> (5.79, -30.0122)
  line L3321 (5.79, -30.0122) -> (5.658, -29.8094)
  line L3322 (5.658, -29.8094) -> (5.5376, -29.6157)
  line L3323 (5.5376, -29.6157) -> (5.4272, -29.4294)
  line L3324 (5.4272, -29.4294) -> (5.3263, -29.2508)
  line L3325 (5.3263, -29.2508) -> (5.2359, -29.0826)
  line L3326 (5.2359, -29.0826) -> (5.1544, -28.9229)
  line L3327 (5.1544, -28.9229) -> (5.0025, -28.6062)
  line L3328 (5.0025, -28.6062) -> (4.9763, -28.5674)
  line L3329 (4.9763, -28.5674) -> (4.951, -28.5421)
  line L3330 (4.951, -28.5421) -> (4.927, -28.5305)
  line L3331 (4.927, -28.5305) -> (4.9104, -28.5306)
  line L3332 (4.9104, -28.5306) -> (4.5288, -28.5936)
  line L3333 (4.5288, -28.5936) -> (4.1464, -28.6516)
  line L3334 (4.1464, -28.6516) -> (4.1305, -28.6567)
  line L3335 (4.1305, -28.6567) -> (4.1114, -28.6751)
  line L3336 (4.1114, -28.6751) -> (4.0951, -28.7069)
  line L3337 (4.0951, -28.7069) -> (4.0822, -28.7519)
  line L3338 (4.0822, -28.7519) -> (4.0356, -29.1001)
  line L3339 (4.0356, -29.1001) -> (4.0074, -29.2771)
  line L3340 (4.0074, -29.2771) -> (3.9734, -29.465)
  line L3341 (3.9734, -29.465) -> (3.9326, -29.6661)
  line L3342 (3.9326, -29.6661) -> (3.8852, -29.8774)
  line L3343 (3.8852, -29.8774) -> (3.8305, -30.0989)
  line L3344 (3.8305, -30.0989) -> (3.7677, -30.3325)
  line L3345 (3.7677, -30.3325) -> (3.6968, -30.5755)
  line L3346 (3.6968, -30.5755) -> (3.6308, -30.7866)
  arc A102 (2.8495, -30.8688) -> (3.6308, -30.7866) centre (0, 0) ccw
  line L3347 (2.8495, -30.8688) -> (2.741, -30.676)
  line L3348 (2.741, -30.676) -> (2.6211, -30.453)
  line L3349 (2.6211, -30.453) -> (2.5111, -30.2376)
  line L3350 (2.5111, -30.2376) -> (2.4116, -30.0323)
  line L3351 (2.4116, -30.0323) -> (2.3213, -29.8355)
  line L3352 (2.3213, -29.8355) -> (2.2396, -29.6473)
  line L3353 (2.2396, -29.6473) -> (2.1673, -29.4705)
  line L3354 (2.1673, -29.4705) -> (2.1029, -29.3033)
  line L3355 (2.1029, -29.3033) -> (1.9849, -28.9724)
  line L3356 (1.9849, -28.9724) -> (1.9629, -28.931)
  line L3357 (1.9629, -28.931) -> (1.9404, -28.9033)
  line L3358 (1.9404, -28.9033) -> (1.9178, -28.8892)
  line L3359 (1.9178, -28.8892) -> (1.9012, -28.8876)
  line L3360 (1.9012, -28.8876) -> (1.5151, -28.9103)
  line L3361 (1.5151, -28.9103) -> (1.1288, -28.9281)
  line L3362 (1.1288, -28.9281) -> (1.1124, -28.9314)
  line L3363 (1.1124, -28.9314) -> (1.0915, -28.9478)
  line L3364 (1.0915, -28.9478) -> (1.0719, -28.9777)
  line L3365 (1.0719, -28.9777) -> (1.0544, -29.0211)
  line L3366 (1.0544, -29.0211) -> (0.9717, -29.3626)
  line L3367 (0.9717, -29.3626) -> (0.9251, -29.5356)
  line L3368 (0.9251, -29.5356) -> (0.8717, -29.719)
  line L3369 (0.8717, -29.719) -> (0.8101, -29.9147)
  line L3370 (0.8101, -29.9147) -> (0.7408, -30.1199)
  line L3371 (0.7408, -30.1199) -> (0.6634, -30.3344)
  line L3372 (0.6634, -30.3344) -> (0.5765, -30.5601)
  line L3373 (0.5765, -30.5601) -> (0.4805, -30.7945)
  line L3374 (0.4805, -30.7945) -> (0.3928, -30.9975)
  arc A103 (-0.3928, -30.9975) -> (0.3928, -30.9975) centre (0, 0) ccw
  line L3375 (-0.3928, -30.9975) -> (-0.4805, -30.7945)
  line L3376 (-0.4805, -30.7945) -> (-0.5765, -30.5601)
  line L3377 (-0.5765, -30.5601) -> (-0.6634, -30.3344)
  line L3378 (-0.6634, -30.3344) -> (-0.7408, -30.1199)
  line L3379 (-0.7408, -30.1199) -> (-0.8101, -29.9147)
  line L3380 (-0.8101, -29.9147) -> (-0.8717, -29.719)
  line L3381 (-0.8717, -29.719) -> (-0.9251, -29.5356)
  line L3382 (-0.9251, -29.5356) -> (-0.9717, -29.3626)
  line L3383 (-0.9717, -29.3626) -> (-1.0544, -29.0211)
  line L3384 (-1.0544, -29.0211) -> (-1.0719, -28.9777)
  line L3385 (-1.0719, -28.9777) -> (-1.0915, -28.9478)
  line L3386 (-1.0915, -28.9478) -> (-1.1124, -28.9314)
  line L3387 (-1.1124, -28.9314) -> (-1.1288, -28.9281)
  line L3388 (-1.1288, -28.9281) -> (-1.5151, -28.9103)
  line L3389 (-1.5151, -28.9103) -> (-1.9012, -28.8876)
  line L3390 (-1.9012, -28.8876) -> (-1.9178, -28.8892)
  line L3391 (-1.9178, -28.8892) -> (-1.9404, -28.9033)
  line L3392 (-1.9404, -28.9033) -> (-1.9629, -28.931)
  line L3393 (-1.9629, -28.931) -> (-1.9849, -28.9724)
  line L3394 (-1.9849, -28.9724) -> (-2.1029, -29.3033)
  line L3395 (-2.1029, -29.3033) -> (-2.1673, -29.4705)
  line L3396 (-2.1673, -29.4705) -> (-2.2396, -29.6473)
  line L3397 (-2.2396, -29.6473) -> (-2.3213, -29.8355)
  line L3398 (-2.3213, -29.8355) -> (-2.4116, -30.0323)
  line L3399 (-2.4116, -30.0323) -> (-2.5111, -30.2376)
  line L3400 (-2.5111, -30.2376) -> (-2.6211, -30.453)
  line L3401 (-2.6211, -30.453) -> (-2.741, -30.676)
  line L3402 (-2.741, -30.676) -> (-2.8495, -30.8688)
  arc A104 (-3.6308, -30.7866) -> (-2.8495, -30.8688) centre (0, 0) ccw
  line L3403 (-3.6308, -30.7866) -> (-3.6968, -30.5755)
  line L3404 (-3.6968, -30.5755) -> (-3.7677, -30.3325)
  line L3405 (-3.7677, -30.3325) -> (-3.8305, -30.0989)
  line L3406 (-3.8305, -30.0989) -> (-3.8852, -29.8774)
  line L3407 (-3.8852, -29.8774) -> (-3.9326, -29.6661)
  line L3408 (-3.9326, -29.6661) -> (-3.9734, -29.465)
  line L3409 (-3.9734, -29.465) -> (-4.0074, -29.2771)
  line L3410 (-4.0074, -29.2771) -> (-4.0356, -29.1001)
  line L3411 (-4.0356, -29.1001) -> (-4.0822, -28.7519)
  line L3412 (-4.0822, -28.7519) -> (-4.0951, -28.7069)
  line L3413 (-4.0951, -28.7069) -> (-4.1114, -28.6751)
  line L3414 (-4.1114, -28.6751) -> (-4.1305, -28.6567)
  line L3415 (-4.1305, -28.6567) -> (-4.1464, -28.6516)
  line L3416 (-4.1464, -28.6516) -> (-4.5288, -28.5936)
  line L3417 (-4.5288, -28.5936) -> (-4.9104, -28.5306)
  line L3418 (-4.9104, -28.5306) -> (-4.927, -28.5305)
  line L3419 (-4.927, -28.5305) -> (-4.951, -28.5421)
  line L3420 (-4.951, -28.5421) -> (-4.9763, -28.5674)
  line L3421 (-4.9763, -28.5674) -> (-5.0025, -28.6062)
  line L3422 (-5.0025, -28.6062) -> (-5.1544, -28.9229)
  line L3423 (-5.1544, -28.9229) -> (-5.2359, -29.0826)
  line L3424 (-5.2359, -29.0826) -> (-5.3263, -29.2508)
  line L3425 (-5.3263, -29.2508) -> (-5.4272, -29.4294)
  line L3426 (-5.4272, -29.4294) -> (-5.5376, -29.6157)
  line L3427 (-5.5376, -29.6157) -> (-5.658, -29.8094)
  line L3428 (-5.658, -29.8094) -> (-5.79, -30.0122)
  line L3429 (-5.79, -30.0122) -> (-5.9325, -30.2214)
  line L3430 (-5.9325, -30.2214) -> (-6.0605, -30.4018)
  arc A105 (-6.829, -30.2385) -> (-6.0605, -30.4018) centre (0, 0) ccw
  line L3431 (-6.829, -30.2385) -> (-6.8726, -30.0216)
  line L3432 (-6.8726, -30.0216) -> (-6.9177, -29.7725)
  line L3433 (-6.9177, -29.7725) -> (-6.9557, -29.5336)
  line L3434 (-6.9557, -29.5336) -> (-6.9869, -29.3077)
  line L3435 (-6.9869, -29.3077) -> (-7.012, -29.0926)
  line L3436 (-7.012, -29.0926) -> (-7.0315, -28.8883)
  line L3437 (-7.0315, -28.8883) -> (-7.0457, -28.6979)
  line L3438 (-7.0457, -28.6979) -> (-7.0553, -28.5189)
  line L3439 (-7.0553, -28.5189) -> (-7.0652, -28.1677)
  line L3440 (-7.0652, -28.1677) -> (-7.0733, -28.1216)
  line L3441 (-7.0733, -28.1216) -> (-7.0862, -28.0883)
  line L3442 (-7.0862, -28.0883) -> (-7.1033, -28.0679)
  line L3443 (-7.1033, -28.0679) -> (-7.1186, -28.0612)
  line L3444 (-7.1186, -28.0612) -> (-7.4928, -27.9636)
  line L3445 (-7.4928, -27.9636) -> (-7.8657, -27.861)
  line L3446 (-7.8657, -27.861) -> (-7.8823, -27.8592)
  line L3447 (-7.8823, -27.8592) -> (-7.9073, -27.8683)
  line L3448 (-7.9073, -27.8683) -> (-7.9351, -27.8907)
  line L3449 (-7.9351, -27.8907) -> (-7.9652, -27.9266)
  line L3450 (-7.9652, -27.9266) -> (-8.1494, -28.2257)
  line L3451 (-8.1494, -28.2257) -> (-8.2472, -28.3759)
  line L3452 (-8.2472, -28.3759) -> (-8.3547, -28.5338)
  line L3453 (-8.3547, -28.5338) -> (-8.4737, -28.7009)
  line L3454 (-8.4737, -28.7009) -> (-8.603, -28.8746)
  line L3455 (-8.603, -28.8746) -> (-8.7429, -29.0547)
  line L3456 (-8.7429, -29.0547) -> (-8.8954, -29.2425)
  line L3457 (-8.8954, -29.2425) -> (-9.059, -29.4358)
  line L3458 (-9.059, -29.4358) -> (-9.2052, -29.6018)
  arc A106 (-9.9523, -29.359) -> (-9.2052, -29.6018) centre (0, 0) ccw
  line L3459 (-9.9523, -29.359) -> (-9.973, -29.1388)
  line L3460 (-9.973, -29.1388) -> (-9.9918, -28.8863)
  line L3461 (-9.9918, -28.8863) -> (-10.0047, -28.6447)
  line L3462 (-10.0047, -28.6447) -> (-10.0121, -28.4168)
  line L3463 (-10.0121, -28.4168) -> (-10.0146, -28.2002)
  line L3464 (-10.0146, -28.2002) -> (-10.0127, -27.995)
  line L3465 (-10.0127, -27.995) -> (-10.0069, -27.8042)
  line L3466 (-10.0069, -27.8042) -> (-9.9977, -27.6252)
  line L3467 (-9.9977, -27.6252) -> (-9.9708, -27.2749)
  line L3468 (-9.9708, -27.2749) -> (-9.9741, -27.2282)
  line L3469 (-9.9741, -27.2282) -> (-9.9834, -27.1937)
  line L3470 (-9.9834, -27.1937) -> (-9.9983, -27.1717)
  line L3471 (-9.9983, -27.1717) -> (-10.0128, -27.1634)
  line L3472 (-10.0128, -27.1634) -> (-10.3748, -27.0272)
  line L3473 (-10.3748, -27.0272) -> (-10.7349, -26.8862)
  line L3474 (-10.7349, -26.8862) -> (-10.7512, -26.8826)
  line L3475 (-10.7512, -26.8826) -> (-10.777, -26.8891)
  line L3476 (-10.777, -26.8891) -> (-10.807, -26.9085)
  line L3477 (-10.807, -26.9085) -> (-10.8407, -26.941)
  line L3478 (-10.8407, -26.941) -> (-11.0551, -27.2193)
  line L3479 (-11.0551, -27.2193) -> (-11.1681, -27.3584)
  line L3480 (-11.1681, -27.3584) -> (-11.2915, -27.5042)
  line L3481 (-11.2915, -27.5042) -> (-11.4273, -27.6579)
  line L3482 (-11.4273, -27.6579) -> (-11.5741, -27.8172)
  line L3483 (-11.5741, -27.8172) -> (-11.7321, -27.9817)
  line L3484 (-11.7321, -27.9817) -> (-11.9033, -28.1525)
  line L3485 (-11.9033, -28.1525) -> (-12.0862, -28.3276)
  line L3486 (-12.0862, -28.3276) -> (-12.249, -28.4774)
  arc A107 (-12.9667, -28.1579) -> (-12.249, -28.4774) centre (0, 0) ccw
  line L3487 (-12.9667, -28.1579) -> (-12.9642, -27.9367)
  line L3488 (-12.9642, -27.9367) -> (-12.9565, -27.6836)
  line L3489 (-12.9565, -27.6836) -> (-12.9441, -27.442)
  line L3490 (-12.9441, -27.442) -> (-12.9276, -27.2145)
  line L3491 (-12.9276, -27.2145) -> (-12.9075, -26.9989)
  line L3492 (-12.9075, -26.9989) -> (-12.8841, -26.7951)
  line L3493 (-12.8841, -26.7951) -> (-12.8584, -26.6059)
  line L3494 (-12.8584, -26.6059) -> (-12.8305, -26.4288)
  line L3495 (-12.8305, -26.4288) -> (-12.7672, -26.0833)
  line L3496 (-12.7672, -26.0833) -> (-12.7656, -26.0365)
  line L3497 (-12.7656, -26.0365) -> (-12.7712, -26.0012)
  line L3498 (-12.7712, -26.0012) -> (-12.7837, -25.9777)
  line L3499 (-12.7837, -25.9777) -> (-12.7973, -25.968)
  line L3500 (-12.7973, -25.968) -> (-13.143, -25.7946)
  line L3501 (-13.143, -25.7946) -> (-13.4865, -25.6168)
  line L3502 (-13.4865, -25.6168) -> (-13.5023, -25.6116)
  line L3503 (-13.5023, -25.6116) -> (-13.5287, -25.6153)
  line L3504 (-13.5287, -25.6153) -> (-13.5605, -25.6314)
  line L3505 (-13.5605, -25.6314) -> (-13.5974, -25.6603)
  line L3506 (-13.5974, -25.6603) -> (-13.8398, -25.9146)
  line L3507 (-13.8398, -25.9146) -> (-13.9666, -26.0412)
  line L3508 (-13.9666, -26.0412) -> (-14.1046, -26.1732)
  line L3509 (-14.1046, -26.1732) -> (-14.2558, -26.312)
  line L3510 (-14.2558, -26.312) -> (-14.4184, -26.455)
  line L3511 (-14.4184, -26.455) -> (-14.5927, -26.602)
  line L3512 (-14.5927, -26.602) -> (-14.7808, -26.7541)
  line L3513 (-14.7808, -26.7541) -> (-14.9811, -26.9091)
  line L3514 (-14.9811, -26.9091) -> (-15.1586, -27.041)
  arc A108 (-15.8389, -26.6482) -> (-15.1586, -27.041) centre (0, 0) ccw
  line L3515 (-15.8389, -26.6482) -> (-15.8134, -26.4285)
  line L3516 (-15.8134, -26.4285) -> (-15.7793, -26.1776)
  line L3517 (-15.7793, -26.1776) -> (-15.7417, -25.9387)
  line L3518 (-15.7417, -25.9387) -> (-15.7015, -25.7142)
  line L3519 (-15.7015, -25.7142) -> (-15.6589, -25.5018)
  line L3520 (-15.6589, -25.5018) -> (-15.6144, -25.3015)
  line L3521 (-15.6144, -25.3015) -> (-15.569, -25.1161)
  line L3522 (-15.569, -25.1161) -> (-15.5228, -24.9429)
  line L3523 (-15.5228, -24.9429) -> (-15.4237, -24.6058)
  line L3524 (-15.4237, -24.6058) -> (-15.4172, -24.5595)
  line L3525 (-15.4172, -24.5595) -> (-15.4191, -24.5238)
  line L3526 (-15.4191, -24.5238) -> (-15.4291, -24.4991)
  line L3527 (-15.4291, -24.4991) -> (-15.4416, -24.488)
  line L3528 (-15.4416, -24.488) -> (-15.7673, -24.2795)
  line L3529 (-15.7673, -24.2795) -> (-16.0903, -24.0668)
  line L3530 (-16.0903, -24.0668) -> (-16.1055, -24.0599)
  line L3531 (-16.1055, -24.0599) -> (-16.1321, -24.0608)
  line L3532 (-16.1321, -24.0608) -> (-16.1655, -24.0735)
  line L3533 (-16.1655, -24.0735) -> (-16.2052, -24.0984)
  line L3534 (-16.2052, -24.0984) -> (-16.4728, -24.326)
  line L3535 (-16.4728, -24.326) -> (-16.6122, -24.4386)
  line L3536 (-16.6122, -24.4386) -> (-16.7632, -24.5555)
  line L3537 (-16.7632, -24.5555) -> (-16.928, -24.6777)
  line L3538 (-16.928, -24.6777) -> (-17.1047, -24.8029)
  line L3539 (-17.1047, -24.8029) -> (-17.2934, -24.931)
  line L3540 (-17.2934, -24.931) -> (-17.4964, -25.0625)
  line L3541 (-17.4964, -25.0625) -> (-17.7118, -25.1957)
  line L3542 (-17.7118, -25.1957) -> (-17.9021, -25.3084)
  arc A109 (-18.5377, -24.8466) -> (-17.9021, -25.3084) centre (0, 0) ccw
  line L3543 (-18.5377, -24.8466) -> (-18.4893, -24.6308)
  line L3544 (-18.4893, -24.6308) -> (-18.4292, -24.3848)
  line L3545 (-18.4292, -24.3848) -> (-18.3668, -24.1511)
  line L3546 (-18.3668, -24.1511) -> (-18.3034, -23.932)
  line L3547 (-18.3034, -23.932) -> (-18.2388, -23.7253)
  line L3548 (-18.2388, -23.7253) -> (-18.1736, -23.5308)
  line L3549 (-18.1736, -23.5308) -> (-18.1091, -23.3511)
  line L3550 (-18.1091, -23.3511) -> (-18.045, -23.1837)
  line L3551 (-18.045, -23.1837) -> (-17.9112, -22.8588)
  line L3552 (-17.9112, -22.8588) -> (-17.8999, -22.8134)
  line L3553 (-17.8999, -22.8134) -> (-17.8981, -22.7777)
  line L3554 (-17.8981, -22.7777) -> (-17.9055, -22.7521)
  line L3555 (-17.9055, -22.7521) -> (-17.9167, -22.7398)
  line L3556 (-17.9167, -22.7398) -> (-18.2188, -22.4984)
  line L3557 (-18.2188, -22.4984) -> (-18.5178, -22.2531)
  line L3558 (-18.5178, -22.2531) -> (-18.5322, -22.2446)
  line L3559 (-18.5322, -22.2446) -> (-18.5587, -22.2427)
  line L3560 (-18.5587, -22.2427) -> (-18.5933, -22.2519)
  line L3561 (-18.5933, -22.2519) -> (-18.6353, -22.2724)
  line L3562 (-18.6353, -22.2724) -> (-18.9253, -22.4708)